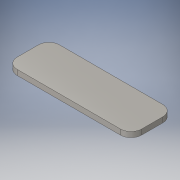
# Autodesk Inventor part: PistonFeederHeadInnerMini
Saved by Autodesk Inventor 2016 (Build 200138000, 138)
## iProperties
Created: 2015-08-02
Part Number: PistonFeederHeadInnerMini
Material: Stainless Steel
Document SubType Name: Modeling
Designer: myhome
Mass: 128.802 g
Surface Area: 91.3119 cm^2
Volume: 16.1002 cm^3
Density: 8 g/cm^3
Appearance: Semi-Polished
Author: myhome
Autodesk Inventor part; units mm, degrees
ref_plane "YZ Plane" through (0, 0, 0) normal (1, 0, 0) x (0, 1, 0)
ref_plane "XZ Plane" through (0, 0, 0) normal (0, 1, 0) x (-1, 0, 0)
ref_plane "XY Plane" through (0, 0, 0) normal (0, 0, 1) x (1, 0, 0)
sketch "Sketch1" plane through (0, 0, 0) normal (0, 0, 1) x (1, 0, 0)
  line L0 (8, 0) -> (86, 0)
  line L1 (94, 8) -> (94, 24)
  line L2 (86, 32) -> (8, 32)
  line L3 (0, 24) -> (0, 8)
  arc A0 (8, 32) -> (0, 24) centre (8, 24) ccw
  arc A1 (94, 24) -> (86, 32) centre (86, 24) ccw
  arc A2 (86, 0) -> (94, 8) centre (86, 8) ccw
  arc A3 (0, 8) -> (8, 0) centre (8, 8) ccw
  circle A4 centre (51, 20) radius 5
  point P0 (0, 0)
  point P1 (94, 32)
  point P2 (94, 0)
  point P3 (0, 32)
  dimension "d0" = 94
  dimension "d1" = 32
  dimension "d2" = 8
  dimension "d3" = 8
  dimension "d6" = 10
  constraints: 8 end point, 8 point on circle, 8 point on line, 8 tangent, 5 centre point, 2 equal radius, 2 parallel, 1 horizontal, 1 perpendicular
  measures "d0" distance of point (94, 32) point (0, 32)
  measures "d1" distance of point (94, 0) point (94, 32)
  measures "d2" radius of A0
  measures "d3" radius of A1
  measures "d6" diameter of A4
extrude "Extrusion1" add sketch "Sketch1" along normal blind 4 contours A3 L3 A0 L2 A1 L1 A2 L0 | A4
body "Solid1"
